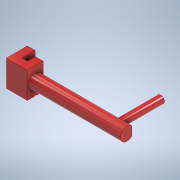
# Autodesk Inventor part: Grip Stopper
Saved by Autodesk Inventor 2020 (Build 240168000, 168)
## iProperties
Created: 2021-06-21
Part Number: Grip Stopper
Material: Generic
Document SubType Name: Modeling
Designer: ugwue
Density: 1 g/cm^3
Appearance: Orange-Red
Author: ugwue
Autodesk Inventor part; units mm, degrees
ref_plane "YZ Plane" through (0, 0, 0) normal (1, 0, 0) x (0, 1, 0)
ref_plane "XZ Plane" through (0, 0, 0) normal (0, 1, 0) x (-1, 0, 0)
ref_plane "XY Plane" through (0, 0, 0) normal (0, 0, 1) x (1, 0, 0)
sketch "Sketch1" plane through (0, 0, 0) normal (0, 0, 1) x (1, 0, 0)
  line L0 (0, 0) -> (8, 0)
  line L1 (8, 0) -> (8, 10)
  line L2 (8, 10) -> (0, 10)
  line L3 (0, 10) -> (0, 0)
  dimension "d0" = 8
  dimension "d1" = 10
  constraints: 8 end point, 2 parallel, 1 horizontal, 1 perpendicular
  measures "d0" distance of L2.end L1.end
  measures "d1" distance of L1.end L0.end
extrude "Extrusion1" add sketch "Sketch1" along normal blind 3
sketch "Sketch2" plane through (8, 0, 0) normal (1, 0, 0) x (0, 0, -1)
  point P0 (0, 0)
sketch "Sketch3" plane through (0, 10, 0) normal (0, 1, 0) x (1, 0, 0)
  line L0 (0, 0) -> (2.95, 0)
  line L1 (2.95, 0) -> (2.95, 5)
  line L2 (2.95, 5) -> (0, 5)
  line L3 (0, 5) -> (0, 0)
  line L4 (8, 0) -> (0, 0) projected
  line L5 (8, 0) -> (8, -3) projected
  line L6 (8, 0) -> (5.05, 0)
  line L7 (5.05, 0) -> (5.05, 3)
  line L8 (5.05, 3) -> (8, 3)
  line L9 (8, 3) -> (8, 0)
  point P0 (5.05, 5)
  dimension "d4" = 2.95
  dimension "d10" = 2.95
  dimension "d11" = 3
  constraints: 16 end point, 4 parallel, 2 horizontal, 2 perpendicular, 1 point on line
  measures "d4" distance of L2.end L1.end
  measures "d10" distance of L7.end L8.end
  measures "d11" distance of L6.end L7.end
extrude "Extrusion2" add sketch "Sketch3" against normal blind 10 contours L3 L2 L1 L0
sketch "Sketch4" plane through (8, 0, 3) normal (1, 0, 0) x (0, 0, -1)
  point P0 (3, 0)
extrude "Extrusion3" add sketch "Sketch3" against normal blind 10 contours L7 L8 L9 L4
sketch "Sketch5" plane through (8, 0, 3) normal (1, 0, 0) x (0, 0, -1)
  line L0 (3, 0) -> (3, 10) projected
  arc A0 (4.8073, 6.7273) -> (4.8073, 3.2727) centre (3, 5) ccw
  line L1 (4.8073, 6.7273) -> (4.8073, 3.2727)
  dimension "d14" = 5
  constraints: 2 end point, 2 point on circle, 1 centre point, 1 midpoint, 1 vertical
  measures "d14" diameter of A0
extrude "Extrusion4" add sketch "Sketch5" along normal blind 35
sketch "Sketch6" plane through (8, 3.2727, -1.8073) normal (0, 0, -1) x (-1, 0, 0)
  line L0 (0, 3.4546) -> (0, 0) projected
  line L1 (0, 1.7273) -> (-30.05, 1.7273)
  circle A0 centre (-30.05, 1.7273) radius 1.45
  point P0 (8, -3.2727)
  dimension "d17" = 30.05
  dimension "d18" = 2.9
  constraints: 2 end point, 1 centre point, 1 coincident, 1 horizontal, 1 midpoint
  measures "d17" distance of L1.start L1.end
  measures "d18" diameter of A0
extrude "Extrusion5" add sketch "Sketch6" along normal blind 16
body "Solid1"
